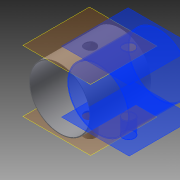
# Autodesk Inventor part: VacuumCylinder
Saved by Autodesk Inventor 2014 (Build 180170000, 170)
## iProperties
Created: 2014-04-15
Part Number: VacuumCylinder
Material: Generic
Document SubType Name: Modeling
Designer: ijs09
Density: 1 g/cm^3
Appearance: Default
Author: ijs09
Autodesk Inventor part; units mm, degrees
ref_plane "YZ Plane" through (0, 0, 0) normal (1, 0, 0) x (0, 1, 0)
ref_plane "XY Plane" through (0, 0, 0) normal (0, 0, 1) x (1, 0, 0)
sketch "Sketch1" plane through (0, 0, 0) normal (0, 0, 1) x (1, 0, 0)
  circle A0 centre (0, 0) radius 98.552
  circle A1 centre (0, 0) radius 101.6
  dimension "d0" = 197.104
  dimension "d1" = 203.2
  constraints: 2 centre point, 2 coincident
  measures "d0" diameter of A0
  measures "d1" diameter of A1
extrude "Extrusion1" add sketch "Sketch1" along normal blind 200
ref_plane "Work Plane1" through (0, 101.6, 0) normal (0, 1, 0) x (-1, 0, 0)
ref_plane "Work Plane2" through (0, -101.6, 0) normal (0, 1, 0) x (-1, 0, 0)
sketch "Sketch7" plane through (0, -101.6, 0) normal (0, 1, 0) x (-1, 0, 0)
  circle A0 centre (0, 100) radius 19
  circle A1 centre (0, 100) radius 20
  line L0 (-101.6, 0) -> (101.6, 0) projected
  point P0 (0, 0)
  point P1 (20, 100)
  dimension "d11" = 40
  dimension "d12" = 38
  dimension "d13" = 100
  constraints: 2 centre point, 1 coincident, 1 other
  measures "d11" diameter of A1
  measures "d12" diameter of A0
  measures "d13" distance from line of A0.centre L0
extrude "Extrusion3" add sketch "Sketch7" along normal up to next
sketch "Sketch9" plane through (0, -101.6, 0) normal (0, 1, 0) x (-1, 0, 0)
  circle A0 centre (0, 100) radius 19
  circle A1 centre (0, 100) radius 20
  point P0 (0, 0)
  point P1 (20, 100)
  dimension "d16" = 40
  dimension "d17" = 38
  constraints: 2 centre point, 1 coincident
  measures "d16" diameter of A1
  measures "d17" diameter of A0
extrude "Extrusion4" add sketch "Sketch9" against normal blind 50
sketch "Sketch10" plane through (0, -101.6, 0) normal (0, 1, 0) x (-1, 0, 0)
  circle A0 centre (0, 100) radius 19
  point P0 (0, 0)
  point P1 (20, 100)
  constraints: 1 centre point
extrude "Extrusion5" cut sketch "Sketch10" along normal through all
equation "\"BendRadius\" = Thickness"
equation "\"BendReliefWidth\" = Thickness"
equation "\"BendReliefDepth\" = 0.5 * Thickness"
equation "\"CornerReliefSize\" = 4 * Thickness"
equation "\"MinimumRemnant\" = 2 * Thickness"
equation "\"TransitionRadius\" = BendRadius"
equation "\"JacobiRadiusSize\" = Thickness"
equation "\"GapSize\" = Thickness"
equation "\"Thickness\" = 3.048"
body "Solid1"
